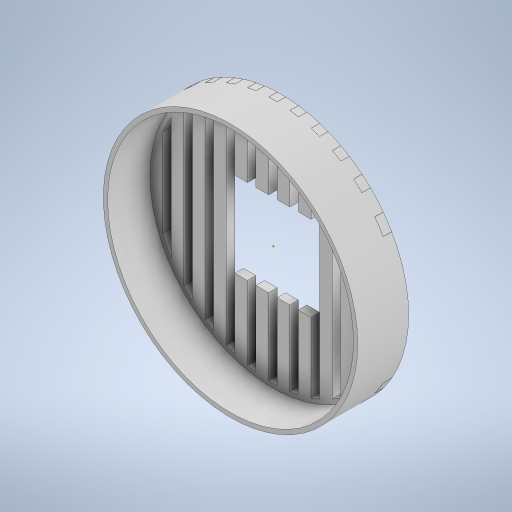
# Autodesk Inventor part: fan back
Saved by Autodesk Inventor 2023.1 (Build 271208000, 208)
## iProperties
Created: 2023-05-29
Part Number: fan back
Material: Generic
Document SubType Name: Modeling
Designer: Mansoor Lunawadi
Density: 1 g/cm^3
Appearance: Default
Author: Mansoor Lunawadi
Autodesk Inventor part; units mm, degrees
ref_plane "YZ Plane" through (0, 0, 0) normal (1, 0, 0) x (0, 1, 0)
ref_plane "XY Plane" through (0, 0, 0) normal (0, 0, 1) x (1, 0, 0)
sketch "Sketch1" plane through (0, 0, 0) normal (0, 0, 1) x (1, 0, 0)
  circle A0 centre (0, 0) radius 30
  dimension "d0" = 60
  constraints: 1 centre point, 1 coincident
  measures "d0" diameter of A0
extrude "Extrusion1" add sketch "Sketch1" against normal blind 10
sketch "Sketch2" plane through (0, 0, -10) normal (0, 0, -1) x (-1, 0, 0)
  circle A0 centre (0, 0) radius 29
  dimension "d3" = 58
  constraints: 1 centre point, 1 coincident
  measures "d3" diameter of A0
extrude "Extrusion2" cut sketch "Sketch2" against normal blind 8
ref_plane "Work Plane1" through (0, 30, 0) normal (0, 1, 0) x (-1, 0, 0)
sketch "Sketch3" plane through (0, 30, 0) normal (0, 1, 0) x (-1, 0, 0)
  line L0 (30, 0) -> (30, -10) projected
  line L1 (30, 0) -> (26, 0)
  line L2 (30, 0) -> (-30, 0) projected
  line L3 (26, 0) -> (24, 0)
  line L4 (24, 0) -> (24, -2)
  line L5 (24, -2) -> (26, -2)
  line L6 (26, -2) -> (26, 0)
  line L7 (24, 0) -> (21, 0)
  line L8 (21, 0) -> (19, 0)
  line L9 (19, 0) -> (19, -2)
  line L10 (19, -2) -> (21, -2)
  line L11 (21, -2) -> (21, 0)
  line L12 (19, 0) -> (16, 0)
  line L13 (16, 0) -> (14, 0)
  line L14 (14, 0) -> (14, -2)
  line L15 (14, -2) -> (16, -2)
  line L16 (16, -2) -> (16, 0)
  line L17 (14, 0) -> (11, 0)
  line L18 (11, 0) -> (9, 0)
  line L19 (9, 0) -> (9, -2)
  line L20 (9, -2) -> (11, -2)
  line L21 (11, -2) -> (11, 0)
  line L22 (9, 0) -> (6, 0)
  line L23 (6, 0) -> (4, 0)
  line L24 (4, 0) -> (4, -2)
  line L25 (4, -2) -> (6, -2)
  line L26 (6, -2) -> (6, 0)
  line L27 (4, 0) -> (1, 0)
  line L28 (1, 0) -> (-1, 0)
  line L29 (-1, 0) -> (-1, -2)
  line L30 (-1, -2) -> (1, -2)
  line L31 (1, -2) -> (1, 0)
  line L32 (-1, 0) -> (-4, 0)
  line L33 (-4, 0) -> (-6, 0)
  line L34 (-6, 0) -> (-6, -2)
  line L35 (-6, -2) -> (-4, -2)
  line L36 (-4, -2) -> (-4, 0)
  line L37 (-6, 0) -> (-9, 0)
  line L38 (-9, 0) -> (-11, 0)
  line L39 (-11, 0) -> (-11, -2)
  line L40 (-11, -2) -> (-9, -2)
  line L41 (-9, -2) -> (-9, 0)
  line L42 (-11, 0) -> (-14, 0)
  line L43 (-14, 0) -> (-16, 0)
  line L44 (-16, 0) -> (-16, -2)
  line L45 (-16, -2) -> (-14, -2)
  line L46 (-14, -2) -> (-14, 0)
  line L47 (-16, 0) -> (-19, 0)
  line L48 (-19, 0) -> (-21, 0)
  line L49 (-21, 0) -> (-21, -2)
  line L50 (-21, -2) -> (-19, -2)
  line L51 (-19, -2) -> (-19, 0)
  line L52 (-21, 0) -> (-24, 0)
  line L53 (-24, 0) -> (-26, 0)
  line L54 (-26, 0) -> (-26, -2)
  line L55 (-26, -2) -> (-24, -2)
  line L56 (-24, -2) -> (-24, 0)
  point P0 (0, 0)
  dimension "d7" = 4
  dimension "d8" = 2
  dimension "d9" = 2
  dimension "d10" = 3
  dimension "d11" = 2
  dimension "d12" = 2
  dimension "d13" = 3
  dimension "d14" = 2
  dimension "d15" = 2
  dimension "d16" = 3
  dimension "d17" = 2
  dimension "d18" = 2
  dimension "d19" = 3
  dimension "d20" = 2
  dimension "d21" = 2
  dimension "d22" = 3
  dimension "d23" = 2
  dimension "d24" = 2
  dimension "d25" = 3
  dimension "d26" = 2
  dimension "d27" = 2
  dimension "d28" = 3
  dimension "d29" = 2
  dimension "d30" = 2
  dimension "d31" = 3
  dimension "d32" = 2
  dimension "d33" = 2
  dimension "d34" = 3
  dimension "d35" = 2
  dimension "d36" = 2
  dimension "d37" = 3
  dimension "d38" = 2
  dimension "d39" = 2
  constraints: 110 end point, 22 parallel, 11 horizontal, 11 perpendicular, 1 point on line, 3 other
  measures "d7" distance of L1.start L1.end
  measures "d8" distance of L5.end L4.end
  measures "d9" distance of L4.end L3.end
  measures "d10" distance of L3.end L7.end
  measures "d11" distance of L10.end L9.end
  measures "d12" distance of L9.end L8.end
  measures "d13" distance of L12.start L16.end
  measures "d14" distance of L15.end L14.end
  measures "d15" distance of L14.end L14.start
  measures "d16" distance of L17.start L21.end
  measures "d17" distance of L20.end L19.end
  measures "d18" distance of L19.end L19.start
  measures "d19" distance of L22.start L26.end
  measures "d20" distance of L25.end L24.end
  measures "d21" distance of L24.end L24.start
  measures "d22" distance of L27.start L31.end
  measures "d23" distance of L30.end L29.end
  measures "d24" distance of L29.end L29.start
  measures "d25" distance of L32.start L36.end
  measures "d26" distance of L35.end L34.end
  measures "d27" distance of L34.end L34.start
  measures "d28" distance of L37.start L41.end
  measures "d29" distance of L40.end L39.end
  measures "d30" distance of L39.end L39.start
  measures "d31" distance of L42.start L46.end
  measures "d32" distance of L45.end L44.end
  measures "d33" distance of L44.end L44.start
  measures "d34" distance of L47.start L51.end
  measures "d35" distance of L50.end L49.end
  measures "d36" distance of L49.end L49.start
  measures "d37" distance of L52.start L56.end
  measures "d38" distance of L55.end L54.end
  measures "d39" distance of L54.end L54.start
extrude "Extrusion3" cut sketch "Sketch3" against normal through all
sketch "Sketch4" plane through (0, 0, -10) normal (0, 0, -1) x (-1, 0, 0)
  circle A0 centre (0, 0) radius 30
  circle A1 centre (0, 0) radius 29
  dimension "d42" = 1
  constraints: 2 centre point, 1 coincident
  measures "d42" radial gap between concentric circles of A0 A1
sketch "Sketch6" plane through (0, 0, 0) normal (1, 0, 0) x (0, 1, 0)
  line L0 (29.9833, 0) -> (29.7321, 0) projected
  line L1 (29.9833, 0) -> (27.9833, 0)
  line L2 (27.9833, 0) -> (27.9833, -2)
  line L3 (27.9833, -2) -> (29.9833, -2)
  line L4 (29.9833, -2) -> (29.9833, 0)
  line L5 (0, -17.9967) -> (0, 37.98) projected
  point P0 (0, 0)
  point P1 (0, 29.9833)
  dimension "d51" = 2
  dimension "d52" = 2
  constraints: 8 end point, 2 parallel, 1 horizontal, 1 perpendicular
  measures "d51" distance of L3.end L2.end
  measures "d52" distance of L2.end L1.end
revolve "Revolution1" add sketch "Sketch6" angle 360 about axis through (0, 0, -10) along (0, 0, 1)
extrude "Extrusion4" cut sketch "Sketch4" against normal blind 8
sketch "Sketch7" plane through (0, 0, 0) normal (0, 0, 1) x (1, 0, 0)
  line L0 (10, 0) -> (20, 0) construction
  line L1 (10, 10) -> (-10, 10)
  line L2 (-10, 10) -> (-10, -10)
  line L3 (-10, -10) -> (10, -10)
  line L4 (10, -10) -> (10, 10)
  point P0 (0, 0)
  dimension "d59" = 10
  dimension "d60" = 10
  dimension "d62" = 20
  dimension "d63" = 20
  constraints: 10 end point, 2 horizontal, 2 parallel, 1 perpendicular
  measures "d59" distance of point (0, 0) L0.start
  measures "d60" distance of L0.start L1.start
  measures "d62" distance of L3.end L2.end
  measures "d63" distance of L2.end L1.end
extrude "Extrusion6" cut sketch "Sketch7" against normal through all
sketch "Sketch9" plane through (0, 0, 0) normal (0, 0, 1) x (1, 0, 0)
  line L0 (19, 23.1948) -> (19, 23.2164) projected
  circle A0 centre (0, 0) radius 30
  circle A1 centre (0, 0) radius 29
  dimension "d68" = 1
  constraints: 1 centre point, 1 coincident, 3 other
extrude "Extrusion8" add sketch "Sketch9" along normal blind 10
body "Solid1"
